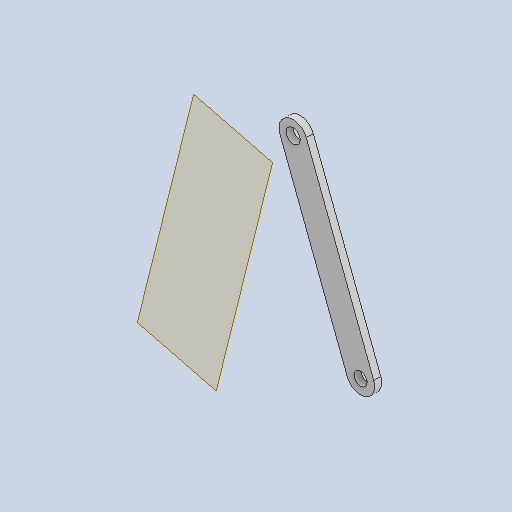
# Autodesk Inventor part: ramieR2
Saved by Autodesk Inventor 2025 (Build 290162000, 162)
## iProperties
Created: 2025-02-05
Part Number: ramieR2
Material: Generic
Document SubType Name: Modeling
Designer: piotr
Density: 1 g/cm^3
Appearance: Default
Author: piotr
Autodesk Inventor part; units mm, degrees
ref_plane "YZ Plane" through (0, 0, 0) normal (1, 0, 0) x (0, 1, 0)
ref_plane "XZ Plane" through (0, 0, 0) normal (0, 1, 0) x (-1, 0, 0)
ref_plane "XY Plane" through (0, 0, 0) normal (0, 0, 1) x (1, 0, 0)
ref_plane "Work Plane1" through (-80.3296, 45.9509, 0) normal (0, 0, 1) x (0.9703, -0.2419, 0)
sketch "Sketch1" plane through (-80.3296, 45.9509, 0) normal (0, 0, 1) x (0.9703, -0.2419, 0)
  arc A0 (244.2307, 28.1499) -> (226.0143, -7.4614) centre (235.1225, 10.3442) ccw projected
  circle A1 centre (235.1225, 10.3442) radius 20 projected
  line L0 (235.1225, 10.3442) -> (81.7542, 230.1217)
  line L1 (473.7181, -111.7057) -> (235.1225, 10.3442) projected
  circle A2 centre (81.7542, 230.1217) radius 20
  circle A3 centre (81.7542, 230.1217) radius 10
  line L2 (65.3529, 218.6763) -> (98.1555, 241.5671)
  line L3 (218.7212, -1.1012) -> (218.7212, -1.1012)
  line L4 (65.3529, 218.6763) -> (98.1555, 241.5671)
  line L5 (98.1555, 241.5671) -> (251.5239, 21.7896)
  line L6 (251.5239, 21.7896) -> (218.7212, -1.1012)
  line L7 (218.7212, -1.1012) -> (65.3529, 218.6763)
  circle A4 centre (235.1225, 10.3442) radius 9.25 projected
  point P0 (89.06, -25.1525)
  point P1 (-51.8234, 125.1812)
  point P2 (-13.0116, 134.8581)
  point P3 (473.7181, -111.7057)
  point P4 (218.7212, -1.1012)
  point P5 (251.5239, 21.7896)
  point P6 (251.5239, 21.7896)
  point P7 (218.7212, -1.1012)
  point P8 (215.3649, 13.448)
  dimension "d0" = 268
  dimension "d1" = 152
  dimension "d2" = 40
  dimension "d3" = 20
  constraints: 14 end point, 3 perpendicular, 2 centre point, 2 coincident, 2 parallel, 2 point on circle, 1 midpoint, 1 point on line, 4 other
  measures "d0" distance of L0.start L0.end
  measures "d2" diameter of A2
  measures "d3" diameter of A3
extrude "Extrusion1" add sketch "Sketch1" along normal blind 10 contours L6 A4 L1 A1 A0 | L7 A2 L0 A0 | A0 L0 A4 L6 | L0 A2 L5 A1 A0 | A0 A1 L6 A4 L0 | L2 A3 L0 A2 | A2 L2 A3 | L1 A4 L6 A1 | L0 A3 L2 A2
body "Solid1"
